Autodesk Inventor part; units mm, degrees
(part 2 of 2)
  circle A60 centre (-42.9331, -32.65) radius 2.5
  circle A61 centre (17, -87.35) radius 2.5
  circle A62 centre (43, -87.35) radius 2.5
  circle A63 centre (-16.9331, -87.35) radius 2.5
  circle A64 centre (-42.9331, -87.35) radius 2.5
  line L258 (0, 94.5) -> (20, 94.5) construction
  line L259 (20, 94.5) -> (-20, 94.5)
  line L260 (-20, 94.5) -> (-20, 111.5)
  line L261 (-20, 111.5) -> (20, 111.5)
  line L262 (20, 111.5) -> (20, 94.5)
  line L263 (0, 0) -> (20, 0) construction
  line L264 (20, 0) -> (-20, 0)
  line L265 (-20, 0) -> (-20, -15)
  line L266 (-20, -15) -> (20, -15)
  line L267 (20, -15) -> (20, 0)
  line L268 (60, -105) -> (60, -15) construction
  line L269 (60, -15) -> (-60, -15) construction
  line L270 (-60, -15) -> (-60, -105) construction
  line L271 (-60, -105) -> (60, -15) construction
  line L272 (60, -105) -> (-60, -15) construction
  line L273 (-72.5, -27.5) -> (-47.5, -27.5)
  line L274 (-47.5, -27.5) -> (-47.5, -2.5)
  line L275 (-47.5, -2.5) -> (-72.5, -2.5)
  line L276 (-72.5, -2.5) -> (-72.5, -27.5)
  line L277 (-72.5, -27.5) -> (-47.5, -2.5) construction
  line L278 (-47.5, -27.5) -> (-72.5, -2.5) construction
  line L279 (47.5, -27.5) -> (72.5, -27.5)
  line L280 (72.5, -27.5) -> (72.5, -2.5)
  line L281 (72.5, -2.5) -> (47.5, -2.5)
  line L282 (47.5, -2.5) -> (47.5, -27.5)
  line L283 (47.5, -27.5) -> (72.5, -2.5) construction
  line L284 (72.5, -27.5) -> (47.5, -2.5) construction
  line L285 (47.5, -117.5) -> (72.5, -117.5)
  line L286 (72.5, -117.5) -> (72.5, -92.5)
  line L287 (72.5, -92.5) -> (47.5, -92.5)
  line L288 (47.5, -92.5) -> (47.5, -117.5)
  line L289 (47.5, -117.5) -> (72.5, -92.5) construction
  line L290 (72.5, -117.5) -> (47.5, -92.5) construction
  line L291 (-72.5, -117.5) -> (-47.5, -117.5)
  line L292 (-47.5, -117.5) -> (-47.5, -92.5)
  line L293 (-47.5, -92.5) -> (-72.5, -92.5)
  line L294 (-72.5, -92.5) -> (-72.5, -117.5)
  line L295 (-72.5, -117.5) -> (-47.5, -92.5) construction
  line L296 (-47.5, -117.5) -> (-72.5, -92.5) construction
  line L297 (43.6642, 136.4728) -> (109.3457, 136.4728) construction
  line L298 (109.3457, 136.4728) -> (109.3457, 114.488) construction
  line L299 (109.3457, 114.488) -> (43.6642, 114.488) construction
  line L300 (43.6642, 114.488) -> (43.6642, 136.4728) construction
  line L301 (-121.8485, 60.4874) -> (-85.7819, 60.4874) construction
  line L302 (-85.7819, 60.4874) -> (-85.7819, 36.8575) construction
  line L303 (-85.7819, 36.8575) -> (-121.8485, 36.8575) construction
  line L304 (-121.8485, 36.8575) -> (-121.8485, 60.4874) construction
  line L305 (100.2542, 65.4138) -> (126.2873, 65.4138) construction
  line L306 (126.2873, 65.4138) -> (126.2873, 51.9268) construction
  line L307 (126.2873, 51.9268) -> (100.2542, 51.9268) construction
  line L308 (100.2542, 51.9268) -> (100.2542, 65.4138) construction
  line L309 (-12.5895, -132.2814) -> (23.7941, -132.2814) construction
  line L310 (23.7941, -132.2814) -> (23.7941, -151.1005) construction
  line L311 (23.7941, -151.1005) -> (-12.5895, -151.1005) construction
  line L312 (-12.5895, -151.1005) -> (-12.5895, -132.2814) construction
  line L313 (-11.9065, 43.812) -> (40.1597, 43.812) construction
  line L314 (40.1597, 43.812) -> (40.1597, 21.5427) construction
  line L315 (40.1597, 21.5427) -> (-11.9065, 21.5427) construction
  line L316 (-11.9065, 21.5427) -> (-11.9065, 43.812) construction
  line L317 (39.4062, -51.8549) -> (69.669, -51.8549) construction
  line L318 (69.669, -51.8549) -> (69.669, -70.0955) construction
  line L319 (69.669, -70.0955) -> (39.4062, -70.0955) construction
  line L320 (39.4062, -70.0955) -> (39.4062, -51.8549) construction
  line L321 (-60.0622, -52.0134) -> (-30.214, -52.0134) construction
  line L322 (-30.214, -52.0134) -> (-30.214, -66.7303) construction
  line L323 (-30.214, -66.7303) -> (-60.0622, -66.7303) construction
  line L324 (-60.0622, -66.7303) -> (-60.0622, -52.0134) construction
  line L325 (-42.75, -175.85) -> (42.75, -175.85) construction
  line L326 (42.75, -175.85) -> (42.75, -119.15) construction
  line L327 (42.75, -119.15) -> (-42.75, -119.15) construction
  line L328 (-42.75, -119.15) -> (-42.75, -175.85) construction
  line L329 (-42.75, -175.85) -> (42.75, -119.15) construction
  line L330 (42.75, -175.85) -> (-42.75, -119.15) construction
  line L331 (-42.75, -119.15) -> (-27.75, -119.15)
  line L332 (-27.75, -119.15) -> (-27.75, -116.15)
  line L333 (-27.75, -116.15) -> (-42.75, -116.15)
  line L334 (-42.75, -116.15) -> (-42.75, -119.15)
  line L335 (42.75, -119.15) -> (27.75, -119.15)
  line L336 (27.75, -119.15) -> (27.75, -116.15)
  line L337 (27.75, -116.15) -> (42.75, -116.15)
  line L338 (42.75, -116.15) -> (42.75, -119.15)
  line L339 (42.75, -116.15) -> (45.75, -116.15)
  line L340 (45.75, -116.15) -> (45.75, -134.15)
  line L341 (45.75, -134.15) -> (42.75, -134.15)
  line L342 (42.75, -134.15) -> (42.75, -116.15)
  line L343 (42.75, -175.85) -> (45.75, -175.85)
  line L344 (45.75, -175.85) -> (45.75, -160.85)
  line L345 (45.75, -160.85) -> (42.75, -160.85)
  line L346 (42.75, -160.85) -> (42.75, -175.85)
  line L347 (45.75, -175.85) -> (27.75, -175.85)
  line L348 (27.75, -175.85) -> (27.75, -178.85)
  line L349 (27.75, -178.85) -> (45.75, -178.85)
  line L350 (45.75, -178.85) -> (45.75, -175.85)
  line L351 (-42.75, -175.85) -> (-27.75, -175.85)
  line L352 (-27.75, -175.85) -> (-27.75, -178.85)
  line L353 (-27.75, -178.85) -> (-42.75, -178.85)
  line L354 (-42.75, -178.85) -> (-42.75, -175.85)
  line L355 (-72, 0) -> (-80.5, 0)
  line L356 (-80.5, 0) -> (-80.5, -3)
  line L357 (-80.5, -3) -> (-72, -3)
  line L358 (-72, -3) -> (-72, 0)
  line L359 (-81, 1) -> (-76, 1)
  line L360 (-76, 1) -> (-76, -0.5)
  line L361 (-76, -0.5) -> (-81, -0.5)
  line L362 (-81, -0.5) -> (-81, 1)
  point P0 (52, -60)
  point P1 (-52, -60)
  point P2 (0, -60)
  point P3 (0, -135)
  point P4 (0, 45)
  point P5 (155.0185, -89.5)
  point P6 (165.4109, -95.5)
  point P7 (89.5, -155.0185)
  point P8 (95.5, -165.4109)
  point P9 (0, -179)
  point P10 (0, -191)
  point P11 (-89.5, -155.0185)
  point P12 (-95.5, -165.4109)
  point P13 (-155.0185, -89.5)
  point P14 (-165.4109, -95.5)
  point P15 (-179, 0)
  point P16 (-191, 0)
  point P17 (-155.0185, 89.5)
  point P18 (-165.4109, 95.5)
  point P19 (-89.5, 155.0185)
  point P20 (-95.5, 165.4109)
  point P21 (0, 179)
  point P22 (0, 191)
  point P23 (89.5, 155.0185)
  point P24 (95.5, 165.4109)
  point P25 (155.0185, 89.5)
  point P26 (165.4109, 95.5)
  dimension "d155" = 350
  dimension "d156" = 390
  dimension "d154" = 400
  dimension "d157" = 50
  dimension "d158" = 114
  dimension "d159" = 50
  dimension "d160" = 200
  dimension "d161" = 96
  dimension "d162" = 96
  dimension "d163" = 42.7
  dimension "d164" = 60
  dimension "d165" = 40
  dimension "d166" = 40
  dimension "d167" = 58
  dimension "d168" = 110
  dimension "d169" = 110
  dimension "d170" = 36.5
  dimension "d171" = 66.5
  dimension "d172" = 42.7
  dimension "d173" = 12
  dimension "d174" = 12
  dimension "d175" = 52
  dimension "d176" = 57.5
  dimension "d177" = 114
  dimension "d178" = 15
  dimension "d179" = 3
  dimension "d180" = 3
  dimension "d181" = 18
  dimension "d182" = 15
  dimension "d183" = 3
  dimension "d184" = 18
  dimension "d185" = 50
  dimension "d186" = 10
  dimension "d187" = 20
  dimension "d188" = 50
  dimension "d189" = 10
  dimension "d190" = 20
  dimension "d191" = 10
  dimension "d192" = 3
  dimension "d193" = 10
  dimension "d194" = 3
  dimension "d195" = 3
  dimension "d196" = 18
  dimension "d197" = 3
  dimension "d198" = 15
  dimension "d199" = 10
  dimension "d200" = 3
  dimension "d201" = 3
  dimension "d202" = 18
  dimension "d203" = 10
  dimension "d204" = 3
  dimension "d205" = 3
  dimension "d206" = 18
  dimension "d207" = 27.3
  dimension "d208" = 27.3
  dimension "d209" = 5
  dimension "d210" = 5
  dimension "d211" = 5
  dimension "d212" = 5
  dimension "d213" = 6
  dimension "d214" = 12
  dimension "d215" = 4
  dimension "d216" = 6
  dimension "d217" = 4
  dimension "d218" = 360
  dimension "d219" = 3
  constraints: 718 end point, 101 parallel, 96 point on circle, 63 centre point, 54 perpendicular, 53 horizontal, 43 midpoint, 28 point on line, 14 coincident, 8 tangent, 3 vertical, 2 horizontal alignment, 1 collinear, 320 other
  measures "d154" diameter of A0
  measures "d157" distance of L1.end L2.end
  measures "d158" distance of L0.end L1.end
  measures "d159" distance of L5.end L6.end
  measures "d160" distance of L8.start L8.end
  measures "d161" distance of L13.start L13.end
  measures "d162" distance of L14.start L14.end
  measures "d163" distance of L16.end L15.end
  measures "d164" distance of L27.start L27.end
  measures "d165" distance of L30.end L29.end
  measures "d166" distance of L29.end L28.end
  measures "d167" distance of L27.start L35.end
  measures "d168" distance of L35.end L36.end
  measures "d169" distance of L35.end L37.end
  measures "d170" distance of L40.end L39.end
  measures "d171" distance of L39.end L38.end
  measures "d172" distance between parallel lines of L21 L23
  measures "d173" distance of L17.end L44.end
  measures "d174" distance of L21.end L45.end
  measures "d175" distance of L66.start L66.end
  measures "d176" distance of L69.end L68.end
  measures "d177" distance of L68.end L67.end
  measures "d178" distance of L75.end L74.end
  measures "d179" distance of L74.end L73.end
  measures "d180" distance of L79.end L78.end
  measures "d181" distance of L78.end L77.end
  measures "d182" distance of L82.end L83.end
  measures "d183" distance of L86.end L87.end
  measures "d184" distance of L85.end L86.end
  measures "d185" distance of L14.start L89.end
  measures "d186" distance of L92.end L91.end
  measures "d187" distance of L91.end L90.end
  measures "d188" distance of L13.start L96.end
  measures "d189" distance of L99.end L98.end
  measures "d190" distance of L98.end L97.end
  measures "d191" distance of L105.end L104.end
  measures "d192" distance of L104.end L103.end
  measures "d193" distance of L108.end L109.end
  measures "d194" distance of L107.end L108.end
  measures "d195" distance of L113.end L112.end
  measures "d196" distance of L112.end L111.end
  measures "d197" distance of L116.end L117.end
  measures "d198" distance of L115.end L116.end
  measures "d199" distance of L120.end L121.end
  measures "d200" distance of L119.end L120.end
  measures "d201" distance of L124.end L125.end
  measures "d202" distance of L123.end L124.end
  measures "d203" distance of L129.end L128.end
  measures "d204" distance of L128.end L127.end
  measures "d205" distance of L133.end L132.end
  measures "d206" distance of L132.end L131.end
  measures "d207" distance of L137.end L136.end
  measures "d208" distance of L136.end L135.end
  measures "d209" diameter of A3
  measures "d210" diameter of A4
  measures "d211" diameter of A5
  measures "d212" diameter of A6
  measures "d213" distance of L142.start L142.end
  measures "d214" distance of L142.end L143.end
  measures "d215" diameter of A8
  measures "d216" distance of L142.start L146.end
  measures "d217" diameter of A10
  measures "d219" distance between parallel lines of L4 L216
extrude "Extrusion7" add sketch "Sketch1" against normal blind 2.5 contours A2 | A4 | A5 | L63 S0 L64 L65 L66 S1 L67 S2 L68 L69 S3 S4 S5 L70 S6 S7 L71 L72 L73 L74 | L77 S9 S8 L76 L75 | L78 L79 L80 L81 S10 S11 S12 L82 S13 L83 L84 L85 L86 L87 S14 S15 S16 L88 L89 L90 L91 L92 S17 S18 L93 L94 L95 L96 S19 S20 L97 S21 L98 L99 L100 L101 | L102 L103 L104 L105 S22 S23 S24 L106 S25 L107 L108 L109 L110 L111 S26 S27 S28 L112 S29 L113 | L114 L115 S30 S31 L116 L117 S32 L118 L119 L120 L121 L122 S33 S34 S35 L123 L124 S36 S37 L125 L126 L127 | L128 L129 L130 S38 L131 S39 S40 L132 S41 S42 L133 L134 L135 L136 S43 S44 L137 S45 S46 S47 L138 S48 L139 | L140 L141 S49 S50 L142 L143 L144 S51 L145 L146 L147 L148 S52 L149 L150 L151 L152 S53 L153 L154 S54 L155 L156 | L157 L158 L159 L160 S55 S56 S57 L161 S58 L162 L163 L164 L165 L166 S59 S60 S61 L167 S62 L168 | L169 S63 S64 L170 L171 L172 S65 L173 L174 L175 L176 S66 S67 S68 L177 L178 S69 S70 S71 L179 L180 | L181 L182 S72 L183 L184 L185 S73 L186 S74 L187 S75 L188 L189 L190 L191 L192 S76 S77 S78 L193 S79 S80 S81 L194 L195 L196 L197 L198 S82 S83 L199 | L200 S84 L201 L202 L203 S85 L204 S86 L205 L206 S87 S88 S89 L207 S90 S91 L208 L209 L210 L211 | L214 S93 S92 L213 L212 | L215 L216 S94 S95 S96 S97 S98 S99 S100 S101 S102 S103 S104 L217 L218 L219 S105 S106 S107 S108 S109 S110 S111 S112 L220 | L221 L222 L223 L224 S113 S114 S115 L225 S116 L226 L227 L228 L229 L230 S117 S118 S119 L231 S120 L232 | L233 L234 S121 S122 L235 L236 S123 L237 L238 L239 L240 L241 S124 S125 S126 L242 L243 S127 S128 L244 L245 L246 | L247 S129 S130 L248 L249 S131 L250 L251 L252 L253 L254 S132 S133 S134 L255 L256 S135 L257 L258 L259 L260 S136 S137 L261 L262 S138 S139 S140 L263 L264
extrude "Extrusion8" add sketch "Sketch1" against normal blind 2.5 contours L32 A3 L31 L30 L29 L28 L27 L26 L25 L24 L23 L22
fillet "Fillet4" radius 1 16 edges at (60, -2, -2.5) (73, -15, -2.5) (47, -15, -2.5) (60, -28, -2.5) (-60, -2, -2.5) (-73, -15, -2.5) (-47, -15, -2.5) (-60, -28, -2.5) (-60, -92, -2.5) (-47, -107.5, -2.5) (-73, -107.5, -2.5) (-60, -123, -2.5) (47, -105, -2.5) (60, -118, -2.5) (73, -105, -2.5) (60, -92, -2.5)
emboss "Emboss2" sketch "Sketch1" operation add depth 1 direction (0, 0, -1) contours L63 S0 L64 L65 L66 S1 L67 S2 L68 L69 S3 S4 S5 L70 S6 S7 L71 L72 L73 L74 | L78 L79 L80 L81 S10 S11 S12 L82 S13 L83 L84 L85 L86 L87 S14 S15 S16 L88 L89 L90 L91 L92 S17 S18 L93 L94 L95 L96 S19 S20 L97 S21 L98 L99 L100 L101 | L102 L103 L104 L105 S22 S23 S24 L106 S25 L107 L108 L109 L110 L111 S26 S27 S28 L112 S29 L113 | L114 L115 S30 S31 L116 L117 S32 L118 L119 L120 L121 L122 S33 S34 S35 L123 L124 S36 S37 L125 L126 L127 | L128 L129 L130 S38 L131 S39 S40 L132 S41 S42 L133 L134 L135 L136 S43 S44 L137 S45 S46 S47 L138 S48 L139 | L140 L141 S49 S50 L142 L143 L144 S51 L145 L146 L147 L148 S52 L149 L150 L151 L152 S53 L153 L154 S54 L155 L156 | L157 L158 L159 L160 S55 S56 S57 L161 S58 L162 L163 L164 L165 L166 S59 S60 S61 L167 S62 L168 | L169 S63 S64 L170 L171 L172 S65 L173 L174 L175 L176 S66 S67 S68 L177 L178 S69 S70 S71 L179 L180 | L181 L182 S72 L183 L184 L185 S73 L186 S74 L187 S75 L188 L189 L190 L191 L192 S76 S77 S78 L193 S79 S80 S81 L194 L195 L196 L197 L198 S82 S83 L199 | L200 S84 L201 L202 L203 S85 L204 S86 L205 L206 S87 S88 S89 L207 S90 S91 L208 L209 L210 L211 | L215 L216 S94 S95 S96 S97 S98 S99 S100 S101 S102 S103 S104 L217 L218 L219 S105 S106 S107 S108 S109 S110 S111 S112 L220 | L221 L222 L223 L224 S113 S114 S115 L225 S116 L226 L227 L228 L229 L230 S117 S118 S119 L231 S120 L232 | L233 L234 S121 S122 L235 L236 S123 L237 L238 L239 L240 L241 S124 S125 S126 L242 L243 S127 S128 L244 L245 L246 | L247 S129 S130 L248 L249 S131 L250 L251 L252 L253 L254 S132 S133 S134 L255 L256 S135 L257 L258 L259 L260 S136 S137 L261 L262 S138 S139 S140 L263 L264
extrude "Extrusion9" add sketch "Sketch1" along normal blind 1 contours A5
body "Solid1"
